Autodesk Inventor part; units mm, degrees
(part 2 of 2)
extrude "Extrusion75" cut sketch "Sketch83" against normal up to surface (142.6892 mm away)
sketch "Sketch84" plane through (105, 94.4392, -39.5005) normal (1, 0, 0) x (0, 0, -1)
  line L0 (0, -104.1392) -> (-23.2505, -104.1392) projected
  line L1 (-79.0007, 10) -> (0, 10) projected
  line L2 (0, -104.1392) -> (-0.828, -104.1392)
  line L3 (-0.828, -104.1392) -> (-0.828, 10)
  line L4 (-0.828, 10) -> (0, 10)
  line L5 (0, 10) -> (0, -104.1392)
  point P0 (-39.5005, -94.4392)
  point P1 (-0.828, -104.1392)
  dimension "d468" = 0.828
  constraints: 8 end point, 2 parallel, 1 horizontal, 1 perpendicular, 1 point on line
  measures "d468" distance between parallel lines of L5 L3
extrude "Extrusion76" cut sketch "Sketch84" against normal up to surface (105 mm away)
sketch "Sketch85" plane through (105, 94.4392, 39.5002) normal (1, 0, 0) x (0, 0, -1)
  line L0 (21.1, -132.6892) -> (0, -132.6892) projected
  line L1 (78.1727, 10) -> (0, 10) projected
  line L2 (0, -132.6892) -> (0.173, -132.6892)
  line L3 (0.173, -132.6892) -> (0.173, 10)
  line L4 (0.173, 10) -> (0, 10)
  line L5 (0, 10) -> (0, -132.6892)
  point P0 (39.5002, -94.4392)
  dimension "d471" = 0.173
  constraints: 8 end point, 2 parallel, 1 horizontal, 1 perpendicular, 1 point on line
  measures "d471" distance between parallel lines of L5 L3
extrude "Extrusion77" cut sketch "Sketch85" against normal up to surface (105 mm away)
sketch "Sketch86" plane through (0, 104.4392, -38.6725) normal (0, 1, 0) x (1, 0, 0)
  circle A0 centre (70, -27.0725) radius 1.5
  circle A1 centre (70, -50.2725) radius 1.5
  circle A2 centre (60, -27.0725) radius 1.5
  circle A3 centre (60, -50.2725) radius 1.5
  circle A4 centre (50, -27.0725) radius 1.5
  circle A5 centre (50, -50.2725) radius 1.5
  line L0 (105, -77.9997) -> (105, 0) projected
  circle A6 centre (40, -27.0725) radius 1.5
  circle A7 centre (40, -50.2725) radius 1.5
  line L1 (0, 0) -> (0, -77.9997) projected
  point P0 (0, -38.6725)
  point P1 (23.9117, -57.7393)
  point P2 (75.0872, -74.2845)
  dimension "d499" = 3
  dimension "d500" = 23.2
  dimension "d501" = 10
  dimension "d502" = 0
  dimension "d503" = 0
  dimension "d504" = 11.6
  dimension "d505" = 10
  dimension "d506" = 0
  dimension "d507" = 0
  dimension "d508" = 0
  dimension "d509" = 35
  dimension "d510" = 10
  dimension "d511" = 10
  dimension "d514" = 10
  dimension "d515" = 10
  dimension "d516" = 23.2
  dimension "d518" = 40
  constraints: 8 centre point, 7 equal radius
  measures "d499" diameter of A3
  measures "d500" distance of A1.centre A0.centre
  measures "d501" distance of A0.centre A2.centre
  measures "d502" vertical distance of A0.centre A2.centre
  measures "d503" vertical distance of A3.centre A1.centre
  measures "d504" vertical distance of A3.centre point (0, -38.672)
  measures "d505" distance of A4.centre A2.centre
  measures "d506" vertical distance of A2.centre A4.centre
  measures "d507" horizontal distance of A4.centre A5.centre
  measures "d508" vertical distance of A3.centre A5.centre
  measures "d509" distance from line of L0 A1.centre
  measures "d510" distance of A1.centre A3.centre
  measures "d511" distance of A3.centre A5.centre
  measures "d514" distance of A6.centre A4.centre
  measures "d515" distance of A5.centre A7.centre
  measures "d516" distance of A6.centre A7.centre
  measures "d518" distance from line of L1 A7.centre
extrude "Extrusion78" cut sketch "Sketch86" against normal blind 10
fillet "Fillet13" radius 2 4 edges at (8, 15.3, 16.25) (8, 15.3, -16.25) (8, -9.7, -16.25) (8, -9.7, 16.25)
chamfer "Chamfer5" distance 1.75 angle 45 18 edges at (16, 2.8, 16.25) (16, -9.1142, 16.8358) (16, -9.7, 18.3251) (16, 14.7142, 15.6642) (16, 15.3, 0) (16, 14.7142, -15.6642) (16, 2.8, -16.25) (16, -9.1142, -16.8358) (16, -9.7, -28.4612) (0, 2.8, 16.25) (0, -9.1142, 16.8358) (0, -9.7, 18.3251) (0, 14.7142, 15.6642) (0, 15.3, 0) (0, 14.7142, -15.6642) (0, 2.8, -16.25) (0, -9.1142, -16.8358) (0, -9.7, -28.4612)
body "Solid1"
